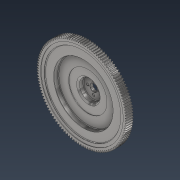
# Autodesk Inventor part: Koło zamachowe poprawione
Saved by Autodesk Inventor 2022 (Build 260153000, 153)
## iProperties
Created: 2023-05-24
Part Number: Koło zamachowe poprawione
Material: Generic
Document SubType Name: Modeling
Designer: wikto
Density: 1 g/cm^3
Appearance: Polished - Small Pyramid Knurl
Author: wikto
Autodesk Inventor part; units mm, degrees
ref_plane "YZ Plane" through (0, 0, 0) normal (1, 0, 0) x (0, 1, 0)
ref_plane "XZ Plane" through (0, 0, 0) normal (0, 1, 0) x (-1, 0, 0)
ref_plane "XY Plane" through (0, 0, 0) normal (0, 0, 1) x (1, 0, 0)
sketch "Sketch2" plane through (0, 0, 20) normal (0, 0, 1) x (0.9945, 0.1045, 0)
  arc A0 (6.9843, 152.34) -> (4.8056, 146.7964) centre (39.556, 136.339) ccw projected
  arc A1 (4.8056, 146.7964) -> (2.8837, 146.8467) centre (0, 0) ccw projected
  arc A2 (2.8837, 146.8467) -> (0.9981, 152.4967) centre (-32.3663, 138.2223) ccw projected
  arc A3 (0.9981, 152.4967) -> (-0.9981, 152.4967) centre (0, 0) ccw projected
  arc A4 (-0.9981, 152.4967) -> (-2.8837, 146.8467) centre (32.3663, 138.2223) ccw projected
  arc A5 (-2.8837, 146.8467) -> (-4.8056, 146.7964) centre (0, 0) ccw projected
  arc A6 (-4.8056, 146.7964) -> (-6.9843, 152.34) centre (-39.556, 136.339) ccw projected
  arc A7 (-6.9843, 152.34) -> (-8.9778, 152.2355) centre (0, 0) ccw projected
  arc A8 (-8.9778, 152.2355) -> (-10.5651, 146.4945) centre (25.088, 139.7268) ccw projected
  arc A9 (-10.5651, 146.4945) -> (-12.4818, 146.3437) centre (0, 0) ccw projected
  arc A10 (-12.4818, 146.3437) -> (-14.9476, 151.7657) centre (-46.6372, 134.0819) ccw projected
  arc A11 (-14.9476, 151.7657) -> (-16.9329, 151.557) centre (0, 0) ccw projected
  arc A12 (-16.9329, 151.557) -> (-18.2176, 145.7408) centre (17.7408, 140.8483) ccw projected
  arc A13 (-18.2176, 145.7408) -> (-20.1237, 145.4899) centre (0, 0) ccw projected
  arc A14 (-20.1237, 145.4899) -> (-22.8699, 150.7754) centre (-53.5906, 131.4574) ccw projected
  arc A15 (-22.8699, 150.7754) -> (-24.8416, 150.4631) centre (0, 0) ccw projected
  arc A16 (-24.8416, 150.4631) -> (-25.8201, 144.5877) centre (10.3451, 141.5838) ccw projected
  arc A17 (-25.8201, 144.5877) -> (-27.7105, 144.2373) centre (0, 0) ccw projected
  arc A18 (-27.7105, 144.2373) -> (-30.7296, 149.3718) centre (-60.3971, 128.4725) ccw projected
  arc A19 (-30.7296, 149.3718) -> (-32.6821, 148.9568) centre (0, 0) ccw projected
  arc A20 (-32.6821, 148.9568) -> (-33.3518, 143.0382) centre (2.921, 141.9312) ccw projected
  arc A21 (-33.3518, 143.0382) -> (-35.2213, 142.5894) centre (0, 0) ccw projected
  arc A22 (-35.2213, 142.5894) -> (-38.505, 147.5589) centre (-67.038, 125.1355) ccw projected
  arc A23 (-38.505, 147.5589) -> (-40.4332, 147.0422) centre (0, 0) ccw projected
  arc A24 (-40.4332, 147.0422) -> (-40.7922, 141.0967) centre (-4.5111, 141.8895) ccw projected
  arc A25 (-40.7922, 141.0967) -> (-42.6356, 140.5506) centre (0, 0) ccw projected
  arc A26 (-42.6356, 140.5506) -> (-46.1748, 145.3414) centre (-73.4952, 121.4555) ccw projected
  arc A27 (-46.1748, 145.3414) -> (-48.0733, 144.7246) centre (0, 0) ccw projected
  arc A28 (-48.0733, 144.7246) -> (-48.1207, 138.7684) centre (-11.9309, 141.459) ccw projected
  arc A29 (-48.1207, 138.7684) -> (-49.933, 138.1266) centre (0, 0) ccw projected
  arc A30 (-49.933, 138.1266) -> (-53.7181, 142.7257) centre (-79.751, 117.4426) ccw projected
  arc A31 (-53.7181, 142.7257) -> (-55.5818, 142.0103) centre (0, 0) ccw projected
  arc A32 (-55.5818, 142.0103) -> (-55.3173, 136.0598) centre (-19.3179, 140.6407) ccw projected
  arc A33 (-55.3173, 136.0598) -> (-57.0935, 135.324) centre (0, 0) ccw projected
  arc A34 (-57.0935, 135.324) -> (-61.1142, 139.7187) centre (-85.7882, 113.1078) ccw projected
  arc A35 (-61.1142, 139.7187) -> (-62.9378, 138.9067) centre (0, 0) ccw projected
  arc A36 (-62.9378, 138.9067) -> (-62.3623, 132.9782) centre (-26.652, 139.4369) ccw projected
  arc A37 (-62.3623, 132.9782) -> (-64.0976, 132.1505) centre (0, 0) ccw projected
  arc A38 (-64.0976, 132.1505) -> (-68.3428, 136.3287) centre (-91.5902, 108.463) ccw projected
  arc A39 (-68.3428, 136.3287) -> (-70.1214, 135.4225) centre (0, 0) ccw projected
  arc A40 (-70.1214, 135.4225) -> (-69.2364, 129.5322) centre (-33.913, 137.851) ccw projected
  arc A41 (-69.2364, 129.5322) -> (-70.926, 128.6148) centre (0, 0) ccw projected
  arc A42 (-70.926, 128.6148) -> (-75.384, 132.5651) centre (-97.1412, 103.5209) ccw projected
  arc A43 (-75.384, 132.5651) -> (-77.1127, 131.567) centre (0, 0) ccw projected
  arc A44 (-77.1127, 131.567) -> (-75.9207, 125.7311) centre (-41.0811, 135.8872) ccw projected
  arc A45 (-75.9207, 125.7311) -> (-77.56, 124.7266) centre (0, 0) ccw projected
  arc A46 (-77.56, 124.7266) -> (-82.2186, 128.4381) centre (-102.426, 98.295) ccw projected
  arc A47 (-82.2186, 128.4381) -> (-83.8928, 127.3509) centre (0, 0) ccw projected
  arc A48 (-83.8928, 127.3509) -> (-82.3969, 121.5854) centre (-48.1366, 133.551) ccw projected
  arc A49 (-82.3969, 121.5854) -> (-83.9814, 120.4965) centre (0, 0) ccw projected
  arc A50 (-83.9814, 120.4965) -> (-88.8278, 123.9591) centre (-107.4299, 92.7998) ccw projected
  arc A51 (-88.8278, 123.9591) -> (-90.4428, 122.7858) centre (0, 0) ccw projected
  arc A52 (-90.4428, 122.7858) -> (-88.6473, 117.1065) centre (-55.0601, 130.8487) ccw projected
  arc A53 (-88.6473, 117.1065) -> (-90.1726, 115.9361) centre (0, 0) ccw projected
  arc A54 (-90.1726, 115.9361) -> (-95.1936, 119.1403) centre (-112.1395, 87.0501) ccw projected
  arc A55 (-95.1936, 119.1403) -> (-96.745, 117.8841) centre (0, 0) ccw projected
  arc A56 (-96.745, 117.8841) -> (-94.6547, 112.3065) centre (-61.8328, 127.7877) ccw projected
  arc A57 (-94.6547, 112.3065) -> (-96.1166, 111.0579) centre (0, 0) ccw projected
  arc A58 (-96.1166, 111.0579) -> (-101.2985, 113.995) centre (-116.5417, 81.0619) ccw projected
  arc A59 (-101.2985, 113.995) -> (-102.782, 112.6593) centre (0, 0) ccw projected
  arc A60 (-102.782, 112.6593) -> (-100.4026, 107.1988) centre (-68.4359, 124.3765) ccw projected
  arc A61 (-100.4026, 107.1988) -> (-101.7972, 105.8754) centre (0, 0) ccw projected
  arc A62 (-101.7972, 105.8754) -> (-107.1257, 108.5372) centre (-120.6244, 74.8515) ccw projected
  arc A63 (-107.1257, 108.5372) -> (-108.5372, 107.1257) centre (0, 0) ccw projected
  arc A64 (-108.5372, 107.1257) -> (-105.8754, 101.7972) centre (-74.8515, 120.6244) ccw projected
  arc A65 (-105.8754, 101.7972) -> (-107.1988, 100.4026) centre (0, 0) ccw projected
  arc A66 (-107.1988, 100.4026) -> (-112.6593, 102.782) centre (-124.3765, 68.4359) ccw projected
  arc A67 (-112.6593, 102.782) -> (-113.995, 101.2985) centre (0, 0) ccw projected
  arc A68 (-113.995, 101.2985) -> (-111.0579, 96.1166) centre (-81.0619, 116.5417) ccw projected
  arc A69 (-111.0579, 96.1166) -> (-112.3065, 94.6547) centre (0, 0) ccw projected
  arc A70 (-112.3065, 94.6547) -> (-117.8841, 96.745) centre (-127.7877, 61.8328) ccw projected
  arc A71 (-117.8841, 96.745) -> (-119.1403, 95.1936) centre (0, 0) ccw projected
  arc A72 (-119.1403, 95.1936) -> (-115.9361, 90.1726) centre (-87.0501, 112.1395) ccw projected
  arc A73 (-115.9361, 90.1726) -> (-117.1065, 88.6473) centre (0, 0) ccw projected
  arc A74 (-117.1065, 88.6473) -> (-122.7858, 90.4428) centre (-130.8487, 55.0601) ccw projected
  arc A75 (-122.7858, 90.4428) -> (-123.9591, 88.8278) centre (0, 0) ccw projected
  arc A76 (-123.9591, 88.8278) -> (-120.4965, 83.9814) centre (-92.7998, 107.4299) ccw projected
  arc A77 (-120.4965, 83.9814) -> (-121.5854, 82.3969) centre (0, 0) ccw projected
  arc A78 (-121.5854, 82.3969) -> (-127.3509, 83.8928) centre (-133.551, 48.1366) ccw projected
  arc A79 (-127.3509, 83.8928) -> (-128.4381, 82.2186) centre (0, 0) ccw projected
  arc A80 (-128.4381, 82.2186) -> (-124.7266, 77.56) centre (-98.295, 102.426) ccw projected
  arc A81 (-124.7266, 77.56) -> (-125.7311, 75.9207) centre (0, 0) ccw projected
  arc A82 (-125.7311, 75.9207) -> (-131.567, 77.1127) centre (-135.8872, 41.0811) ccw projected
  arc A83 (-131.567, 77.1127) -> (-132.5651, 75.384) centre (0, 0) ccw projected
  arc A84 (-132.5651, 75.384) -> (-128.6148, 70.926) centre (-103.5209, 97.1412) ccw projected
  arc A85 (-128.6148, 70.926) -> (-129.5322, 69.2364) centre (0, 0) ccw projected
  arc A86 (-129.5322, 69.2364) -> (-135.4225, 70.1214) centre (-137.851, 33.913) ccw projected
  arc A87 (-135.4225, 70.1214) -> (-136.3287, 68.3428) centre (0, 0) ccw projected
  arc A88 (-136.3287, 68.3428) -> (-132.1505, 64.0976) centre (-108.463, 91.5902) ccw projected
  arc A89 (-132.1505, 64.0976) -> (-132.9782, 62.3623) centre (0, 0) ccw projected
  arc A90 (-132.9782, 62.3623) -> (-138.9067, 62.9378) centre (-139.4369, 26.652) ccw projected
  arc A91 (-138.9067, 62.9378) -> (-139.7187, 61.1142) centre (0, 0) ccw projected
  arc A92 (-139.7187, 61.1142) -> (-135.324, 57.0935) centre (-113.1078, 85.7882) ccw projected
  arc A93 (-135.324, 57.0935) -> (-136.0598, 55.3173) centre (0, 0) ccw projected
  arc A94 (-136.0598, 55.3173) -> (-142.0103, 55.5818) centre (-140.6407, 19.3179) ccw projected
  arc A95 (-142.0103, 55.5818) -> (-142.7257, 53.7181) centre (0, 0) ccw projected
  arc A96 (-142.7257, 53.7181) -> (-138.1266, 49.933) centre (-117.4426, 79.751) ccw projected
  arc A97 (-138.1266, 49.933) -> (-138.7684, 48.1207) centre (0, 0) ccw projected
  arc A98 (-138.7684, 48.1207) -> (-144.7246, 48.0733) centre (-141.459, 11.9309) ccw projected
  arc A99 (-144.7246, 48.0733) -> (-145.3414, 46.1748) centre (0, 0) ccw projected
  arc A100 (-145.3414, 46.1748) -> (-140.5506, 42.6356) centre (-121.4555, 73.4952) ccw projected
  arc A101 (-140.5506, 42.6356) -> (-141.0967, 40.7922) centre (0, 0) ccw projected
  arc A102 (-141.0967, 40.7922) -> (-147.0422, 40.4332) centre (-141.8895, 4.5111) ccw projected
  arc A103 (-147.0422, 40.4332) -> (-147.5589, 38.505) centre (0, 0) ccw projected
  arc A104 (-147.5589, 38.505) -> (-142.5894, 35.2213) centre (-125.1355, 67.038) ccw projected
  arc A105 (-142.5894, 35.2213) -> (-143.0382, 33.3518) centre (0, 0) ccw projected
  arc A106 (-143.0382, 33.3518) -> (-148.9568, 32.6821) centre (-141.9312, -2.921) ccw projected
  arc A107 (-148.9568, 32.6821) -> (-149.3718, 30.7296) centre (0, 0) ccw projected
  arc A108 (-149.3718, 30.7296) -> (-144.2373, 27.7105) centre (-128.4725, 60.3971) ccw projected
  arc A109 (-144.2373, 27.7105) -> (-144.5877, 25.8201) centre (0, 0) ccw projected
  arc A110 (-144.5877, 25.8201) -> (-150.4631, 24.8416) centre (-141.5838, -10.3451) ccw projected
  arc A111 (-150.4631, 24.8416) -> (-150.7754, 22.8699) centre (0, 0) ccw projected
  arc A112 (-150.7754, 22.8699) -> (-145.4899, 20.1237) centre (-131.4574, 53.5906) ccw projected
  arc A113 (-145.4899, 20.1237) -> (-145.7408, 18.2176) centre (0, 0) ccw projected
  arc A114 (-145.7408, 18.2176) -> (-151.557, 16.9329) centre (-140.8483, -17.7408) ccw projected
  arc A115 (-151.557, 16.9329) -> (-151.7657, 14.9476) centre (0, 0) ccw projected
  arc A116 (-151.7657, 14.9476) -> (-146.3437, 12.4818) centre (-134.0819, 46.6372) ccw projected
  arc A117 (-146.3437, 12.4818) -> (-146.4945, 10.5651) centre (0, 0) ccw projected
  arc A118 (-146.4945, 10.5651) -> (-152.2355, 8.9778) centre (-139.7268, -25.088) ccw projected
  arc A119 (-152.2355, 8.9778) -> (-152.34, 6.9843) centre (0, 0) ccw projected
  arc A120 (-152.34, 6.9843) -> (-146.7964, 4.8056) centre (-136.339, 39.556) ccw projected
  arc A121 (-146.7964, 4.8056) -> (-146.8467, 2.8837) centre (0, 0) ccw projected
  arc A122 (-146.8467, 2.8837) -> (-152.4967, 0.9981) centre (-138.2223, -32.3663) ccw projected
  arc A123 (-152.4967, 0.9981) -> (-152.4967, -0.9981) centre (0, 0) ccw projected
  arc A124 (-152.4967, -0.9981) -> (-146.8467, -2.8837) centre (-138.2223, 32.3663) ccw projected
  arc A125 (-146.8467, -2.8837) -> (-146.7964, -4.8056) centre (0, 0) ccw projected
  arc A126 (-146.7964, -4.8056) -> (-152.34, -6.9843) centre (-136.339, -39.556) ccw projected
  arc A127 (-152.34, -6.9843) -> (-152.2355, -8.9778) centre (0, 0) ccw projected
  arc A128 (-152.2355, -8.9778) -> (-146.4945, -10.5651) centre (-139.7268, 25.088) ccw projected
  arc A129 (-146.4945, -10.5651) -> (-146.3437, -12.4818) centre (0, 0) ccw projected
  arc A130 (-146.3437, -12.4818) -> (-151.7657, -14.9476) centre (-134.0819, -46.6372) ccw projected
  arc A131 (-151.7657, -14.9476) -> (-151.557, -16.9329) centre (0, 0) ccw projected
  arc A132 (-151.557, -16.9329) -> (-145.7408, -18.2176) centre (-140.8483, 17.7408) ccw projected
  arc A133 (-145.7408, -18.2176) -> (-145.4899, -20.1237) centre (0, 0) ccw projected
  arc A134 (-145.4899, -20.1237) -> (-150.7754, -22.8699) centre (-131.4574, -53.5906) ccw projected
  arc A135 (-150.7754, -22.8699) -> (-150.4631, -24.8416) centre (0, 0) ccw projected
  arc A136 (-150.4631, -24.8416) -> (-144.5877, -25.8201) centre (-141.5838, 10.3451) ccw projected
  arc A137 (-144.5877, -25.8201) -> (-144.2373, -27.7105) centre (0, 0) ccw projected
  arc A138 (-144.2373, -27.7105) -> (-149.3718, -30.7296) centre (-128.4725, -60.3971) ccw projected
  arc A139 (-149.3718, -30.7296) -> (-148.9568, -32.6821) centre (0, 0) ccw projected
  arc A140 (-148.9568, -32.6821) -> (-143.0382, -33.3518) centre (-141.9312, 2.921) ccw projected
  arc A141 (-143.0382, -33.3518) -> (-142.5894, -35.2213) centre (0, 0) ccw projected
  arc A142 (-142.5894, -35.2213) -> (-147.5589, -38.505) centre (-125.1355, -67.038) ccw projected
  arc A143 (-147.5589, -38.505) -> (-147.0422, -40.4332) centre (0, 0) ccw projected
  arc A144 (-147.0422, -40.4332) -> (-141.0967, -40.7922) centre (-141.8895, -4.5111) ccw projected
  arc A145 (-141.0967, -40.7922) -> (-140.5506, -42.6356) centre (0, 0) ccw projected
  arc A146 (-140.5506, -42.6356) -> (-145.3414, -46.1748) centre (-121.4555, -73.4952) ccw projected
  arc A147 (-145.3414, -46.1748) -> (-144.7246, -48.0733) centre (0, 0) ccw projected
  arc A148 (-144.7246, -48.0733) -> (-138.7684, -48.1207) centre (-141.459, -11.9309) ccw projected
  arc A149 (-138.7684, -48.1207) -> (-138.1266, -49.933) centre (0, 0) ccw projected
  arc A150 (-138.1266, -49.933) -> (-142.7257, -53.7181) centre (-117.4426, -79.751) ccw projected
  arc A151 (-142.7257, -53.7181) -> (-142.0103, -55.5818) centre (0, 0) ccw projected
  arc A152 (-142.0103, -55.5818) -> (-136.0598, -55.3173) centre (-140.6407, -19.3179) ccw projected
  arc A153 (-136.0598, -55.3173) -> (-135.324, -57.0935) centre (0, 0) ccw projected
  arc A154 (-135.324, -57.0935) -> (-139.7187, -61.1142) centre (-113.1078, -85.7882) ccw projected
  arc A155 (-139.7187, -61.1142) -> (-138.9067, -62.9378) centre (0, 0) ccw projected
  arc A156 (-138.9067, -62.9378) -> (-132.9782, -62.3623) centre (-139.4369, -26.652) ccw projected
  arc A157 (-132.9782, -62.3623) -> (-132.1505, -64.0976) centre (0, 0) ccw projected
  arc A158 (-132.1505, -64.0976) -> (-136.3287, -68.3428) centre (-108.463, -91.5902) ccw projected
  arc A159 (-136.3287, -68.3428) -> (-135.4225, -70.1214) centre (0, 0) ccw projected
  arc A160 (-135.4225, -70.1214) -> (-129.5322, -69.2364) centre (-137.851, -33.913) ccw projected
  arc A161 (-129.5322, -69.2364) -> (-128.6148, -70.926) centre (0, 0) ccw projected
  arc A162 (-128.6148, -70.926) -> (-132.5651, -75.384) centre (-103.5209, -97.1412) ccw projected
  arc A163 (-132.5651, -75.384) -> (-131.567, -77.1127) centre (0, 0) ccw projected
  arc A164 (-131.567, -77.1127) -> (-125.7311, -75.9207) centre (-135.8872, -41.0811) ccw projected
  arc A165 (-125.7311, -75.9207) -> (-124.7266, -77.56) centre (0, 0) ccw projected
  arc A166 (-124.7266, -77.56) -> (-128.4381, -82.2186) centre (-98.295, -102.426) ccw projected
  arc A167 (-128.4381, -82.2186) -> (-127.3509, -83.8928) centre (0, 0) ccw projected
  arc A168 (-127.3509, -83.8928) -> (-121.5854, -82.3969) centre (-133.551, -48.1366) ccw projected
  arc A169 (-121.5854, -82.3969) -> (-120.4965, -83.9814) centre (0, 0) ccw projected
  arc A170 (-120.4965, -83.9814) -> (-123.9591, -88.8278) centre (-92.7998, -107.4299) ccw projected
  arc A171 (-123.9591, -88.8278) -> (-122.7858, -90.4428) centre (0, 0) ccw projected
  arc A172 (-122.7858, -90.4428) -> (-117.1065, -88.6473) centre (-130.8487, -55.0601) ccw projected
  arc A173 (-117.1065, -88.6473) -> (-115.9361, -90.1726) centre (0, 0) ccw projected
  arc A174 (-115.9361, -90.1726) -> (-119.1403, -95.1936) centre (-87.0501, -112.1395) ccw projected
  arc A175 (-119.1403, -95.1936) -> (-117.8841, -96.745) centre (0, 0) ccw projected
  arc A176 (-117.8841, -96.745) -> (-112.3065, -94.6547) centre (-127.7877, -61.8328) ccw projected
  arc A177 (-112.3065, -94.6547) -> (-111.0579, -96.1166) centre (0, 0) ccw projected
  arc A178 (-111.0579, -96.1166) -> (-113.995, -101.2985) centre (-81.0619, -116.5417) ccw projected
  arc A179 (-113.995, -101.2985) -> (-112.6593, -102.782) centre (0, 0) ccw projected
  arc A180 (-112.6593, -102.782) -> (-107.1988, -100.4026) centre (-124.3765, -68.4359) ccw projected
  arc A181 (-107.1988, -100.4026) -> (-105.8754, -101.7972) centre (0, 0) ccw projected
  arc A182 (-105.8754, -101.7972) -> (-108.5372, -107.1257) centre (-74.8515, -120.6244) ccw projected
  arc A183 (-108.5372, -107.1257) -> (-107.1257, -108.5372) centre (0, 0) ccw projected
  arc A184 (-107.1257, -108.5372) -> (-101.7972, -105.8754) centre (-120.6244, -74.8515) ccw projected
  arc A185 (-101.7972, -105.8754) -> (-100.4026, -107.1988) centre (0, 0) ccw projected
  arc A186 (-100.4026, -107.1988) -> (-102.782, -112.6593) centre (-68.4359, -124.3765) ccw projected
  arc A187 (-102.782, -112.6593) -> (-101.2985, -113.995) centre (0, 0) ccw projected
  arc A188 (-101.2985, -113.995) -> (-96.1166, -111.0579) centre (-116.5417, -81.0619) ccw projected
  arc A189 (-96.1166, -111.0579) -> (-94.6547, -112.3065) centre (0, 0) ccw projected
  arc A190 (-94.6547, -112.3065) -> (-96.745, -117.8841) centre (-61.8328, -127.7877) ccw projected
  arc A191 (-96.745, -117.8841) -> (-95.1936, -119.1403) centre (0, 0) ccw projected
  arc A192 (-95.1936, -119.1403) -> (-90.1726, -115.9361) centre (-112.1395, -87.0501) ccw projected
  arc A193 (-90.1726, -115.9361) -> (-88.6473, -117.1065) centre (0, 0) ccw projected
  arc A194 (-88.6473, -117.1065) -> (-90.4428, -122.7858) centre (-55.0601, -130.8487) ccw projected
  arc A195 (-90.4428, -122.7858) -> (-88.8278, -123.9591) centre (0, 0) ccw projected
  arc A196 (-88.8278, -123.9591) -> (-83.9814, -120.4965) centre (-107.4299, -92.7998) ccw projected
  arc A197 (-83.9814, -120.4965) -> (-82.3969, -121.5854) centre (0, 0) ccw projected
  arc A198 (-82.3969, -121.5854) -> (-83.8928, -127.3509) centre (-48.1366, -133.551) ccw projected
  arc A199 (-83.8928, -127.3509) -> (-82.2186, -128.4381) centre (0, 0) ccw projected
  arc A200 (-82.2186, -128.4381) -> (-77.56, -124.7266) centre (-102.426, -98.295) ccw projected
  arc A201 (-77.56, -124.7266) -> (-75.9207, -125.7311) centre (0, 0) ccw projected
  arc A202 (-75.9207, -125.7311) -> (-77.1127, -131.567) centre (-41.0811, -135.8872) ccw projected
  arc A203 (-77.1127, -131.567) -> (-75.384, -132.5651) centre (0, 0) ccw projected
  arc A204 (-75.384, -132.5651) -> (-70.926, -128.6148) centre (-97.1412, -103.5209) ccw projected
  arc A205 (-70.926, -128.6148) -> (-69.2364, -129.5322) centre (0, 0) ccw projected
  arc A206 (-69.2364, -129.5322) -> (-70.1214, -135.4225) centre (-33.913, -137.851) ccw projected
  arc A207 (-70.1214, -135.4225) -> (-68.3428, -136.3287) centre (0, 0) ccw projected
  arc A208 (-68.3428, -136.3287) -> (-64.0976, -132.1505) centre (-91.5902, -108.463) ccw projected
  arc A209 (-64.0976, -132.1505) -> (-62.3623, -132.9782) centre (0, 0) ccw projected
  arc A210 (-62.3623, -132.9782) -> (-62.9378, -138.9067) centre (-26.652, -139.4369) ccw projected
  arc A211 (-62.9378, -138.9067) -> (-61.1142, -139.7187) centre (0, 0) ccw projected
  arc A212 (-61.1142, -139.7187) -> (-57.0935, -135.324) centre (-85.7882, -113.1078) ccw projected
  arc A213 (-57.0935, -135.324) -> (-55.3173, -136.0598) centre (0, 0) ccw projected
  arc A214 (-55.3173, -136.0598) -> (-55.5818, -142.0103) centre (-19.3179, -140.6407) ccw projected
  arc A215 (-55.5818, -142.0103) -> (-53.7181, -142.7257) centre (0, 0) ccw projected
  arc A216 (-53.7181, -142.7257) -> (-49.933, -138.1266) centre (-79.751, -117.4426) ccw projected
  arc A217 (-49.933, -138.1266) -> (-48.1207, -138.7684) centre (0, 0) ccw projected
  arc A218 (-48.1207, -138.7684) -> (-48.0733, -144.7246) centre (-11.9309, -141.459) ccw projected
  arc A219 (-48.0733, -144.7246) -> (-46.1748, -145.3414) centre (0, 0) ccw projected
  arc A220 (-46.1748, -145.3414) -> (-42.6356, -140.5506) centre (-73.4952, -121.4555) ccw projected
  arc A221 (-42.6356, -140.5506) -> (-40.7922, -141.0967) centre (0, 0) ccw projected
  arc A222 (-40.7922, -141.0967) -> (-40.4332, -147.0422) centre (-4.5111, -141.8895) ccw projected
  arc A223 (-40.4332, -147.0422) -> (-38.505, -147.5589) centre (0, 0) ccw projected
  arc A224 (-38.505, -147.5589) -> (-35.2213, -142.5894) centre (-67.038, -125.1355) ccw projected
  arc A225 (-35.2213, -142.5894) -> (-33.3518, -143.0382) centre (0, 0) ccw projected
  arc A226 (-33.3518, -143.0382) -> (-32.6821, -148.9568) centre (2.921, -141.9312) ccw projected
  arc A227 (-32.6821, -148.9568) -> (-30.7296, -149.3718) centre (0, 0) ccw projected
  arc A228 (-30.7296, -149.3718) -> (-27.7105, -144.2373) centre (-60.3971, -128.4725) ccw projected
  arc A229 (-27.7105, -144.2373) -> (-25.8201, -144.5877) centre (0, 0) ccw projected
  arc A230 (-25.8201, -144.5877) -> (-24.8416, -150.4631) centre (10.3451, -141.5838) ccw projected
  arc A231 (-24.8416, -150.4631) -> (-22.8699, -150.7754) centre (0, 0) ccw projected
  arc A232 (-22.8699, -150.7754) -> (-20.1237, -145.4899) centre (-53.5906, -131.4574) ccw projected
  arc A233 (-20.1237, -145.4899) -> (-18.2176, -145.7408) centre (0, 0) ccw projected
  arc A234 (-18.2176, -145.7408) -> (-16.9329, -151.557) centre (17.7408, -140.8483) ccw projected
  arc A235 (-16.9329, -151.557) -> (-14.9476, -151.7657) centre (0, 0) ccw projected
  arc A236 (-14.9476, -151.7657) -> (-12.4818, -146.3437) centre (-46.6372, -134.0819) ccw projected
  arc A237 (-12.4818, -146.3437) -> (-10.5651, -146.4945) centre (0, 0) ccw projected
  arc A238 (-10.5651, -146.4945) -> (-8.9778, -152.2355) centre (25.088, -139.7268) ccw projected
  arc A239 (-8.9778, -152.2355) -> (-6.9843, -152.34) centre (0, 0) ccw projected
  arc A240 (-6.9843, -152.34) -> (-4.8056, -146.7964) centre (-39.556, -136.339) ccw projected
  arc A241 (-4.8056, -146.7964) -> (-2.8837, -146.8467) centre (0, 0) ccw projected
  arc A242 (-2.8837, -146.8467) -> (-0.9981, -152.4967) centre (32.3663, -138.2223) ccw projected
  arc A243 (-0.9981, -152.4967) -> (0.9981, -152.4967) centre (0, 0) ccw projected
  arc A244 (0.9981, -152.4967) -> (2.8837, -146.8467) centre (-32.3663, -138.2223) ccw projected
  arc A245 (2.8837, -146.8467) -> (4.8056, -146.7964) centre (0, 0) ccw projected
  arc A246 (4.8056, -146.7964) -> (6.9843, -152.34) centre (39.556, -136.339) ccw projected
  arc A247 (6.9843, -152.34) -> (8.9778, -152.2355) centre (0, 0) ccw projected
  arc A248 (8.9778, -152.2355) -> (10.5651, -146.4945) centre (-25.088, -139.7268) ccw projected
  arc A249 (10.5651, -146.4945) -> (12.4818, -146.3437) centre (0, 0) ccw projected
  arc A250 (12.4818, -146.3437) -> (14.9476, -151.7657) centre (46.6372, -134.0819) ccw projected
  arc A251 (14.9476, -151.7657) -> (16.9329, -151.557) centre (0, 0) ccw projected
  arc A252 (16.9329, -151.557) -> (18.2176, -145.7408) centre (-17.7408, -140.8483) ccw projected
  arc A253 (18.2176, -145.7408) -> (20.1237, -145.4899) centre (0, 0) ccw projected
  arc A254 (20.1237, -145.4899) -> (22.8699, -150.7754) centre (53.5906, -131.4574) ccw projected
  arc A255 (22.8699, -150.7754) -> (24.8416, -150.4631) centre (0, 0) ccw projected
  arc A256 (24.8416, -150.4631) -> (25.8201, -144.5877) centre (-10.3451, -141.5838) ccw projected
  arc A257 (25.8201, -144.5877) -> (27.7105, -144.2373) centre (0, 0) ccw projected
  arc A258 (27.7105, -144.2373) -> (30.7296, -149.3718) centre (60.3971, -128.4725) ccw projected
  arc A259 (30.7296, -149.3718) -> (32.6821, -148.9568) centre (0, 0) ccw projected
  arc A260 (32.6821, -148.9568) -> (33.3518, -143.0382) centre (-2.921, -141.9312) ccw projected
  arc A261 (33.3518, -143.0382) -> (35.2213, -142.5894) centre (0, 0) ccw projected
  arc A262 (35.2213, -142.5894) -> (38.505, -147.5589) centre (67.038, -125.1355) ccw projected
  arc A263 (38.505, -147.5589) -> (40.4332, -147.0422) centre (0, 0) ccw projected
  arc A264 (40.4332, -147.0422) -> (40.7922, -141.0967) centre (4.5111, -141.8895) ccw projected
  arc A265 (40.7922, -141.0967) -> (42.6356, -140.5506) centre (0, 0) ccw projected
  arc A266 (42.6356, -140.5506) -> (46.1748, -145.3414) centre (73.4952, -121.4555) ccw projected
  arc A267 (46.1748, -145.3414) -> (48.0733, -144.7246) centre (0, 0) ccw projected
  arc A268 (48.0733, -144.7246) -> (48.1207, -138.7684) centre (11.9309, -141.459) ccw projected
  arc A269 (48.1207, -138.7684) -> (49.933, -138.1266) centre (0, 0) ccw projected
  arc A270 (49.933, -138.1266) -> (53.7181, -142.7257) centre (79.751, -117.4426) ccw projected
  arc A271 (53.7181, -142.7257) -> (55.5818, -142.0103) centre (0, 0) ccw projected
  arc A272 (55.5818, -142.0103) -> (55.3173, -136.0598) centre (19.3179, -140.6407) ccw projected
  arc A273 (55.3173, -136.0598) -> (57.0935, -135.324) centre (0, 0) ccw projected
  arc A274 (57.0935, -135.324) -> (61.1142, -139.7187) centre (85.7882, -113.1078) ccw projected
  arc A275 (61.1142, -139.7187) -> (62.9378, -138.9067) centre (0, 0) ccw projected
  arc A276 (62.9378, -138.9067) -> (62.3623, -132.9782) centre (26.652, -139.4369) ccw projected
  arc A277 (62.3623, -132.9782) -> (64.0976, -132.1505) centre (0, 0) ccw projected
  arc A278 (64.0976, -132.1505) -> (68.3428, -136.3287) centre (91.5902, -108.463) ccw projected
  arc A279 (68.3428, -136.3287) -> (70.1214, -135.4225) centre (0, 0) ccw projected
  arc A280 (70.1214, -135.4225) -> (69.2364, -129.5322) centre (33.913, -137.851) ccw projected
  arc A281 (69.2364, -129.5322) -> (70.926, -128.6148) centre (0, 0) ccw projected
  arc A282 (70.926, -128.6148) -> (75.384, -132.5651) centre (97.1412, -103.5209) ccw projected
  arc A283 (75.384, -132.5651) -> (77.1127, -131.567) centre (0, 0) ccw projected
  arc A284 (77.1127, -131.567) -> (75.9207, -125.7311) centre (41.0811, -135.8872) ccw projected
  arc A285 (75.9207, -125.7311) -> (77.56, -124.7266) centre (0, 0) ccw projected
  arc A286 (77.56, -124.7266) -> (82.2186, -128.4381) centre (102.426, -98.295) ccw projected
  arc A287 (82.2186, -128.4381) -> (83.8928, -127.3509) centre (0, 0) ccw projected
  arc A288 (83.8928, -127.3509) -> (82.3969, -121.5854) centre (48.1366, -133.551) ccw projected
  arc A289 (82.3969, -121.5854) -> (83.9814, -120.4965) centre (0, 0) ccw projected
  arc A290 (83.9814, -120.4965) -> (88.8278, -123.9591) centre (107.4299, -92.7998) ccw projected
  arc A291 (88.8278, -123.9591) -> (90.4428, -122.7858) centre (0, 0) ccw projected
  arc A292 (90.4428, -122.7858) -> (88.6473, -117.1065) centre (55.0601, -130.8487) ccw projected
  arc A293 (88.6473, -117.1065) -> (90.1726, -115.9361) centre (0, 0) ccw projected
  arc A294 (90.1726, -115.9361) -> (95.1936, -119.1403) centre (112.1395, -87.0501) ccw projected
  arc A295 (95.1936, -119.1403) -> (96.745, -117.8841) centre (0, 0) ccw projected
  arc A296 (96.745, -117.8841) -> (94.6547, -112.3065) centre (61.8328, -127.7877) ccw projected
  arc A297 (94.6547, -112.3065) -> (96.1166, -111.0579) centre (0, 0) ccw projected
  arc A298 (96.1166, -111.0579) -> (101.2985, -113.995) centre (116.5417, -81.0619) ccw projected
  arc A299 (101.2985, -113.995) -> (102.782, -112.6593) centre (0, 0) ccw projected
  arc A300 (102.782, -112.6593) -> (100.4026, -107.1988) centre (68.4359, -124.3765) ccw projected
  arc A301 (100.4026, -107.1988) -> (101.7972, -105.8754) centre (0, 0) ccw projected
  arc A302 (101.7972, -105.8754) -> (107.1257, -108.5372) centre (120.6244, -74.8515) ccw projected
  arc A303 (107.1257, -108.5372) -> (108.5372, -107.1257) centre (0, 0) ccw projected
  arc A304 (108.5372, -107.1257) -> (105.8754, -101.7972) centre (74.8515, -120.6244) ccw projected
  arc A305 (105.8754, -101.7972) -> (107.1988, -100.4026) centre (0, 0) ccw projected
  arc A306 (107.1988, -100.4026) -> (112.6593, -102.782) centre (124.3765, -68.4359) ccw projected
  arc A307 (112.6593, -102.782) -> (113.995, -101.2985) centre (0, 0) ccw projected
  arc A308 (113.995, -101.2985) -> (111.0579, -96.1166) centre (81.0619, -116.5417) ccw projected
  arc A309 (111.0579, -96.1166) -> (112.3065, -94.6547) centre (0, 0) ccw projected
  arc A310 (112.3065, -94.6547) -> (117.8841, -96.745) centre (127.7877, -61.8328) ccw projected
  arc A311 (117.8841, -96.745) -> (119.1403, -95.1936) centre (0, 0) ccw projected
  arc A312 (119.1403, -95.1936) -> (115.9361, -90.1726) centre (87.0501, -112.1395) ccw projected
  arc A313 (115.9361, -90.1726) -> (117.1065, -88.6473) centre (0, 0) ccw projected
  arc A314 (117.1065, -88.6473) -> (122.7858, -90.4428) centre (130.8487, -55.0601) ccw projected
  arc A315 (122.7858, -90.4428) -> (123.9591, -88.8278) centre (0, 0) ccw projected
  arc A316 (123.9591, -88.8278) -> (120.4965, -83.9814) centre (92.7998, -107.4299) ccw projected
  arc A317 (120.4965, -83.9814) -> (121.5854, -82.3969) centre (0, 0) ccw projected
  arc A318 (121.5854, -82.3969) -> (127.3509, -83.8928) centre (133.551, -48.1366) ccw projected
  arc A319 (127.3509, -83.8928) -> (128.4381, -82.2186) centre (0, 0) ccw projected
  arc A320 (128.4381, -82.2186) -> (124.7266, -77.56) centre (98.295, -102.426) ccw projected
  arc A321 (124.7266, -77.56) -> (125.7311, -75.9207) centre (0, 0) ccw projected
  arc A322 (125.7311, -75.9207) -> (131.567, -77.1127) centre (135.8872, -41.0811) ccw projected
  arc A323 (131.567, -77.1127) -> (132.5651, -75.384) centre (0, 0) ccw projected
  arc A324 (132.5651, -75.384) -> (128.6148, -70.926) centre (103.5209, -97.1412) ccw projected
  arc A325 (128.6148, -70.926) -> (129.5322, -69.2364) centre (0, 0) ccw projected
  arc A326 (129.5322, -69.2364) -> (135.4225, -70.1214) centre (137.851, -33.913) ccw projected
  arc A327 (135.4225, -70.1214) -> (136.3287, -68.3428) centre (0, 0) ccw projected
  arc A328 (136.3287, -68.3428) -> (132.1505, -64.0976) centre (108.463, -91.5902) ccw projected
  arc A329 (132.1505, -64.0976) -> (132.9782, -62.3623) centre (0, 0) ccw projected
  arc A330 (132.9782, -62.3623) -> (138.9067, -62.9378) centre (139.4369, -26.652) ccw projected
  arc A331 (138.9067, -62.9378) -> (139.7187, -61.1142) centre (0, 0) ccw projected
  arc A332 (139.7187, -61.1142) -> (135.324, -57.0935) centre (113.1078, -85.7882) ccw projected
  arc A333 (135.324, -57.0935) -> (136.0598, -55.3173) centre (0, 0) ccw projected
  arc A334 (136.0598, -55.3173) -> (142.0103, -55.5818) centre (140.6407, -19.3179) ccw projected
  arc A335 (142.0103, -55.5818) -> (142.7257, -53.7181) centre (0, 0) ccw projected
  arc A336 (142.7257, -53.7181) -> (138.1266, -49.933) centre (117.4426, -79.751) ccw projected
  arc A337 (138.1266, -49.933) -> (138.7684, -48.1207) centre (0, 0) ccw projected
  arc A338 (138.7684, -48.1207) -> (144.7246, -48.0733) centre (141.459, -11.9309) ccw projected
  arc A339 (144.7246, -48.0733) -> (145.3414, -46.1748) centre (0, 0) ccw projected
  arc A340 (145.3414, -46.1748) -> (140.5506, -42.6356) centre (121.4555, -73.4952) ccw projected
  arc A341 (140.5506, -42.6356) -> (141.0967, -40.7922) centre (0, 0) ccw projected
  arc A342 (141.0967, -40.7922) -> (147.0422, -40.4332) centre (141.8895, -4.5111) ccw projected
  arc A343 (147.0422, -40.4332) -> (147.5589, -38.505) centre (0, 0) ccw projected
  arc A344 (147.5589, -38.505) -> (142.5894, -35.2213) centre (125.1355, -67.038) ccw projected
  arc A345 (142.5894, -35.2213) -> (143.0382, -33.3518) centre (0, 0) ccw projected
  arc A346 (143.0382, -33.3518) -> (148.9568, -32.6821) centre (141.9312, 2.921) ccw projected
  arc A347 (148.9568, -32.6821) -> (149.3718, -30.7296) centre (0, 0) ccw projected
  arc A348 (149.3718, -30.7296) -> (144.2373, -27.7105) centre (128.4725, -60.3971) ccw projected
  arc A349 (144.2373, -27.7105) -> (144.5877, -25.8201) centre (0, 0) ccw projected
  arc A350 (144.5877, -25.8201) -> (150.4631, -24.8416) centre (141.5838, 10.3451) ccw projected
  arc A351 (150.4631, -24.8416) -> (150.7754, -22.8699) centre (0, 0) ccw projected
  arc A352 (150.7754, -22.8699) -> (145.4899, -20.1237) centre (131.4574, -53.5906) ccw projected
  arc A353 (145.4899, -20.1237) -> (145.7408, -18.2176) centre (0, 0) ccw projected
  arc A354 (145.7408, -18.2176) -> (151.557, -16.9329) centre (140.8483, 17.7408) ccw projected
  arc A355 (151.557, -16.9329) -> (151.7657, -14.9476) centre (0, 0) ccw projected
  arc A356 (151.7657, -14.9476) -> (146.3437, -12.4818) centre (134.0819, -46.6372) ccw projected
  arc A357 (146.3437, -12.4818) -> (146.4945, -10.5651) centre (0, 0) ccw projected
  arc A358 (146.4945, -10.5651) -> (152.2355, -8.9778) centre (139.7268, 25.088) ccw projected
  arc A359 (152.2355, -8.9778) -> (152.34, -6.9843) centre (0, 0) ccw projected
  arc A360 (152.34, -6.9843) -> (146.7964, -4.8056) centre (136.339, -39.556) ccw projected
  arc A361 (146.7964, -4.8056) -> (146.8467, -2.8837) centre (0, 0) ccw projected
  arc A362 (146.8467, -2.8837) -> (152.4967, -0.9981) centre (138.2223, 32.3663) ccw projected
  arc A363 (152.4967, -0.9981) -> (152.4967, 0.9981) centre (0, 0) ccw projected
  arc A364 (152.4967, 0.9981) -> (146.8467, 2.8837) centre (138.2223, -32.3663) ccw projected
  arc A365 (146.8467, 2.8837) -> (146.7964, 4.8056) centre (0, 0) ccw projected
  arc A366 (146.7964, 4.8056) -> (152.34, 6.9843) centre (136.339, 39.556) ccw projected
  arc A367 (152.34, 6.9843) -> (152.2355, 8.9778) centre (0, 0) ccw projected
  arc A368 (152.2355, 8.9778) -> (146.4945, 10.5651) centre (139.7268, -25.088) ccw projected
  arc A369 (146.4945, 10.5651) -> (146.3437, 12.4818) centre (0, 0) ccw projected
  arc A370 (146.3437, 12.4818) -> (151.7657, 14.9476) centre (134.0819, 46.6372) ccw projected
  arc A371 (151.7657, 14.9476) -> (151.557, 16.9329) centre (0, 0) ccw projected
  arc A372 (151.557, 16.9329) -> (145.7408, 18.2176) centre (140.8483, -17.7408) ccw projected
  arc A373 (145.7408, 18.2176) -> (145.4899, 20.1237) centre (0, 0) ccw projected
  arc A374 (145.4899, 20.1237) -> (150.7754, 22.8699) centre (131.4574, 53.5906) ccw projected
  arc A375 (150.7754, 22.8699) -> (150.4631, 24.8416) centre (0, 0) ccw projected
  arc A376 (150.4631, 24.8416) -> (144.5877, 25.8201) centre (141.5838, -10.3451) ccw projected
  arc A377 (144.5877, 25.8201) -> (144.2373, 27.7105) centre (0, 0) ccw projected
  arc A378 (144.2373, 27.7105) -> (149.3718, 30.7296) centre (128.4725, 60.3971) ccw projected
  arc A379 (149.3718, 30.7296) -> (148.9568, 32.6821) centre (0, 0) ccw projected
  arc A380 (148.9568, 32.6821) -> (143.0382, 33.3518) centre (141.9312, -2.921) ccw projected
  arc A381 (143.0382, 33.3518) -> (142.5894, 35.2213) centre (0, 0) ccw projected
  arc A382 (142.5894, 35.2213) -> (147.5589, 38.505) centre (125.1355, 67.038) ccw projected
  arc A383 (147.5589, 38.505) -> (147.0422, 40.4332) centre (0, 0) ccw projected
  arc A384 (147.0422, 40.4332) -> (141.0967, 40.7922) centre (141.8895, 4.5111) ccw projected
  arc A385 (141.0967, 40.7922) -> (140.5506, 42.6356) centre (0, 0) ccw projected
  arc A386 (140.5506, 42.6356) -> (145.3414, 46.1748) centre (121.4555, 73.4952) ccw projected
  arc A387 (145.3414, 46.1748) -> (144.7246, 48.0733) centre (0, 0) ccw projected
  arc A388 (144.7246, 48.0733) -> (138.7684, 48.1207) centre (141.459, 11.9309) ccw projected
  arc A389 (138.7684, 48.1207) -> (138.1266, 49.933) centre (0, 0) ccw projected
  arc A390 (138.1266, 49.933) -> (142.7257, 53.7181) centre (117.4426, 79.751) ccw projected
  arc A391 (142.7257, 53.7181) -> (142.0103, 55.5818) centre (0, 0) ccw projected
  arc A392 (142.0103, 55.5818) -> (136.0598, 55.3173) centre (140.6407, 19.3179) ccw projected
  arc A393 (136.0598, 55.3173) -> (135.324, 57.0935) centre (0, 0) ccw projected
  arc A394 (135.324, 57.0935) -> (139.7187, 61.1142) centre (113.1078, 85.7882) ccw projected
  arc A395 (139.7187, 61.1142) -> (138.9067, 62.9378) centre (0, 0) ccw projected
  arc A396 (138.9067, 62.9378) -> (132.9782, 62.3623) centre (139.4369, 26.652) ccw projected
  arc A397 (132.9782, 62.3623) -> (132.1505, 64.0976) centre (0, 0) ccw projected
  arc A398 (132.1505, 64.0976) -> (136.3287, 68.3428) centre (108.463, 91.5902) ccw projected
  arc A399 (136.3287, 68.3428) -> (135.4225, 70.1214) centre (0, 0) ccw projected
  arc A400 (135.4225, 70.1214) -> (129.5322, 69.2364) centre (137.851, 33.913) ccw projected
  arc A401 (129.5322, 69.2364) -> (128.6148, 70.926) centre (0, 0) ccw projected
  arc A402 (128.6148, 70.926) -> (132.5651, 75.384) centre (103.5209, 97.1412) ccw projected
  arc A403 (132.5651, 75.384) -> (131.567, 77.1127) centre (0, 0) ccw projected
  arc A404 (131.567, 77.1127) -> (125.7311, 75.9207) centre (135.8872, 41.0811) ccw projected
  arc A405 (125.7311, 75.9207) -> (124.7266, 77.56) centre (0, 0) ccw projected
  arc A406 (124.7266, 77.56) -> (128.4381, 82.2186) centre (98.295, 102.426) ccw projected
  arc A407 (128.4381, 82.2186) -> (127.3509, 83.8928) centre (0, 0) ccw projected
  arc A408 (127.3509, 83.8928) -> (121.5854, 82.3969) centre (133.551, 48.1366) ccw projected
  arc A409 (121.5854, 82.3969) -> (120.4965, 83.9814) centre (0, 0) ccw projected
  arc A410 (120.4965, 83.9814) -> (123.9591, 88.8278) centre (92.7998, 107.4299) ccw projected
  arc A411 (123.9591, 88.8278) -> (122.7858, 90.4428) centre (0, 0) ccw projected
  arc A412 (122.7858, 90.4428) -> (117.1065, 88.6473) centre (130.8487, 55.0601) ccw projected
  arc A413 (117.1065, 88.6473) -> (115.9361, 90.1726) centre (0, 0) ccw projected
  arc A414 (115.9361, 90.1726) -> (119.1403, 95.1936) centre (87.0501, 112.1395) ccw projected
  arc A415 (119.1403, 95.1936) -> (117.8841, 96.745) centre (0, 0) ccw projected
  arc A416 (117.8841, 96.745) -> (112.3065, 94.6547) centre (127.7877, 61.8328) ccw projected
  arc A417 (112.3065, 94.6547) -> (111.0579, 96.1166) centre (0, 0) ccw projected
  arc A418 (111.0579, 96.1166) -> (113.995, 101.2985) centre (81.0619, 116.5417) ccw projected
  arc A419 (113.995, 101.2985) -> (112.6593, 102.782) centre (0, 0) ccw projected
  arc A420 (112.6593, 102.782) -> (107.1988, 100.4026) centre (124.3765, 68.4359) ccw projected
  arc A421 (107.1988, 100.4026) -> (105.8754, 101.7972) centre (0, 0) ccw projected
  arc A422 (105.8754, 101.7972) -> (108.5372, 107.1257) centre (74.8515, 120.6244) ccw projected
  arc A423 (108.5372, 107.1257) -> (107.1257, 108.5372) centre (0, 0) ccw projected
  arc A424 (107.1257, 108.5372) -> (101.7972, 105.8754) centre (120.6244, 74.8515) ccw projected
  arc A425 (101.7972, 105.8754) -> (100.4026, 107.1988) centre (0, 0) ccw projected
  arc A426 (100.4026, 107.1988) -> (102.782, 112.6593) centre (68.4359, 124.3765) ccw projected
  arc A427 (102.782, 112.6593) -> (101.2985, 113.995) centre (0, 0) ccw projected
  arc A428 (101.2985, 113.995) -> (96.1166, 111.0579) centre (116.5417, 81.0619) ccw projected
  arc A429 (96.1166, 111.0579) -> (94.6547, 112.3065) centre (0, 0) ccw projected
  arc A430 (94.6547, 112.3065) -> (96.745, 117.8841) centre (61.8328, 127.7877) ccw projected
  arc A431 (96.745, 117.8841) -> (95.1936, 119.1403) centre (0, 0) ccw projected
  arc A432 (95.1936, 119.1403) -> (90.1726, 115.9361) centre (112.1395, 87.0501) ccw projected
  arc A433 (90.1726, 115.9361) -> (88.6473, 117.1065) centre (0, 0) ccw projected
  arc A434 (88.6473, 117.1065) -> (90.4428, 122.7858) centre (55.0601, 130.8487) ccw projected
  arc A435 (90.4428, 122.7858) -> (88.8278, 123.9591) centre (0, 0) ccw projected
  arc A436 (88.8278, 123.9591) -> (83.9814, 120.4965) centre (107.4299, 92.7998) ccw projected
  arc A437 (83.9814, 120.4965) -> (82.3969, 121.5854) centre (0, 0) ccw projected
  arc A438 (82.3969, 121.5854) -> (83.8928, 127.3509) centre (48.1366, 133.551) ccw projected
  arc A439 (83.8928, 127.3509) -> (82.2186, 128.4381) centre (0, 0) ccw projected
  arc A440 (82.2186, 128.4381) -> (77.56, 124.7266) centre (102.426, 98.295) ccw projected
  arc A441 (77.56, 124.7266) -> (75.9207, 125.7311) centre (0, 0) ccw projected
  arc A442 (75.9207, 125.7311) -> (77.1127, 131.567) centre (41.0811, 135.8872) ccw projected
  arc A443 (77.1127, 131.567) -> (75.384, 132.5651) centre (0, 0) ccw projected
  arc A444 (75.384, 132.5651) -> (70.926, 128.6148) centre (97.1412, 103.5209) ccw projected
  arc A445 (70.926, 128.6148) -> (69.2364, 129.5322) centre (0, 0) ccw projected
  arc A446 (69.2364, 129.5322) -> (70.1214, 135.4225) centre (33.913, 137.851) ccw projected
  arc A447 (70.1214, 135.4225) -> (68.3428, 136.3287) centre (0, 0) ccw projected
  arc A448 (68.3428, 136.3287) -> (64.0976, 132.1505) centre (91.5902, 108.463) ccw projected
  arc A449 (64.0976, 132.1505) -> (62.3623, 132.9782) centre (0, 0) ccw projected
  arc A450 (62.3623, 132.9782) -> (62.9378, 138.9067) centre (26.652, 139.4369) ccw projected
  arc A451 (62.9378, 138.9067) -> (61.1142, 139.7187) centre (0, 0) ccw projected
  arc A452 (61.1142, 139.7187) -> (57.0935, 135.324) centre (85.7882, 113.1078) ccw projected
  arc A453 (57.0935, 135.324) -> (55.3173, 136.0598) centre (0, 0) ccw projected
  arc A454 (55.3173, 136.0598) -> (55.5818, 142.0103) centre (19.3179, 140.6407) ccw projected
  arc A455 (55.5818, 142.0103) -> (53.7181, 142.7257) centre (0, 0) ccw projected
  arc A456 (53.7181, 142.7257) -> (49.933, 138.1266) centre (79.751, 117.4426) ccw projected
  arc A457 (49.933, 138.1266) -> (48.1207, 138.7684) centre (0, 0) ccw projected
  arc A458 (48.1207, 138.7684) -> (48.0733, 144.7246) centre (11.9309, 141.459) ccw projected
  arc A459 (48.0733, 144.7246) -> (46.1748, 145.3414) centre (0, 0) ccw projected
  arc A460 (46.1748, 145.3414) -> (42.6356, 140.5506) centre (73.4952, 121.4555) ccw projected
  arc A461 (42.6356, 140.5506) -> (40.7922, 141.0967) centre (0, 0) ccw projected
  arc A462 (40.7922, 141.0967) -> (40.4332, 147.0422) centre (4.5111, 141.8895) ccw projected
  arc A463 (40.4332, 147.0422) -> (38.505, 147.5589) centre (0, 0) ccw projected
  arc A464 (38.505, 147.5589) -> (35.2213, 142.5894) centre (67.038, 125.1355) ccw projected
  arc A465 (35.2213, 142.5894) -> (33.3518, 143.0382) centre (0, 0) ccw projected
  arc A466 (33.3518, 143.0382) -> (32.6821, 148.9568) centre (-2.921, 141.9312) ccw projected
  arc A467 (32.6821, 148.9568) -> (30.7296, 149.3718) centre (0, 0) ccw projected
  arc A468 (30.7296, 149.3718) -> (27.7105, 144.2373) centre (60.3971, 128.4725) ccw projected
  arc A469 (27.7105, 144.2373) -> (25.8201, 144.5877) centre (0, 0) ccw projected
  arc A470 (25.8201, 144.5877) -> (24.8416, 150.4631) centre (-10.3451, 141.5838) ccw projected
  arc A471 (24.8416, 150.4631) -> (22.8699, 150.7754) centre (0, 0) ccw projected
  arc A472 (22.8699, 150.7754) -> (20.1237, 145.4899) centre (53.5906, 131.4574) ccw projected
  arc A473 (20.1237, 145.4899) -> (18.2176, 145.7408) centre (0, 0) ccw projected
  arc A474 (18.2176, 145.7408) -> (16.9329, 151.557) centre (-17.7408, 140.8483) ccw projected
  arc A475 (16.9329, 151.557) -> (14.9476, 151.7657) centre (0, 0) ccw projected
  arc A476 (14.9476, 151.7657) -> (12.4818, 146.3437) centre (46.6372, 134.0819) ccw projected
  arc A477 (12.4818, 146.3437) -> (10.5651, 146.4945) centre (0, 0) ccw projected
  arc A478 (10.5651, 146.4945) -> (8.9778, 152.2355) centre (-25.088, 139.7268) ccw projected
  arc A479 (8.9778, 152.2355) -> (6.9843, 152.34) centre (0, 0) ccw projected
extrude "Extrusion1" add sketch "Sketch2" against normal blind 50
sketch "Sketch1" plane through (0, 0, 20) normal (0, 0, 1) x (0.9945, 0.1045, 0)
  circle A0 centre (0, 0) radius 140
  circle A1 centre (0, 0) radius 130
  circle A2 centre (0, 0) radius 100
  circle A3 centre (0, 0) radius 65
  circle A4 centre (0, 0) radius 35
  circle A5 centre (0, 0) radius 14.15
  dimension "d1" = 280
  dimension "d2" = 260
  dimension "d3" = 200
  dimension "d4" = 28.3
  dimension "d5" = 70
  dimension "d6" = 130
  constraints: 6 centre point, 6 coincident
  measures "d1" diameter of A0
  measures "d2" diameter of A1
  measures "d3" diameter of A2
  measures "d4" diameter of A5
  measures "d5" diameter of A4
  measures "d6" diameter of A3
extrude "Extrusion2" cut sketch "Sketch1" against normal blind 2 contours A0 | A1 | A2 | A3 | A4 | A5
extrude "Extrusion3" cut sketch "Sketch1" against normal blind 5 contours A1 | A2 | A3 | A4 | A5
extrude "Extrusion4" cut sketch "Sketch1" against normal blind 20 contours A2 | A3 | A4 | A5
extrude "Extrusion5" cut sketch "Sketch1" against normal blind 22 contours A3 | A4 | A5
extrude "Extrusion6" cut sketch "Sketch1" against normal through all contours A5
extrude "Extrusion7" cut sketch "Sketch1" against normal blind 40 contours A4 | A5
sketch "Sketch3" plane through (0, 0, -20) normal (0, 0, 1) x (1, 0, 0)
  circle A0 centre (0, 0) radius 20.5
  point P0 (0, 20.5)
  point P1 (-20.5, 0)
  point P2 (0, -20.5)
  point P3 (20.5, 0)
  dimension "d21" = 41
  dimension "d24" = 360
  constraints: 2 vertical alignment, 1 coincident, 7 other
hole "Hole1" at (0, 20.5, -20) at (-20.5, 0, -20) at (0, -20.5, -20) at (20.5, 0, -20) direction (0, 0, -1) diameter 8 end through all
chamfer "Chamfer1" distance 5 angle 45 1 edges at (-34.8083, -3.6585, -2)
fillet "Fillet1" radius 2 3 edges at (-34.8083, -3.6585, -20) (-99.4522, -10.4528, 0) (-129.2878, -13.5887, 15)
chamfer "Chamfer2" distance 1 angle 45 1 edges at (-99.4522, -10.4528, 15)
sketch "Sketch4" plane through (0, 0, -30) normal (0, 0, -1) x (-0.9945, -0.1045, 0)
  circle A0 centre (0, 0) radius 27.5
  circle A1 centre (0, 0) radius 35
  dimension "d40" = 55
  dimension "d41" = 70
  constraints: 2 centre point, 2 coincident
  measures "d40" diameter of A0
  measures "d41" diameter of A1
extrude "Extrusion8" add sketch "Sketch4" along normal blind 5
sketch "Sketch5" plane through (0, 0, -30) normal (0, 0, -1) x (-0.9945, -0.1045, 0)
  circle A0 centre (0, 0) radius 35 projected
  circle A1 centre (0, 0) radius 140 projected
  circle A2 centre (0, 0) radius 14.15 projected
  circle A3 centre (0, 0) radius 155
  circle A4 centre (0, 0) radius 127.5
  circle A5 centre (0, 0) radius 75
  circle A6 centre (0, 0) radius 12.5
  dimension "d44" = 310
  dimension "d45" = 255
  dimension "d46" = 150
  dimension "d61" = 25
  constraints: 4 centre point, 4 coincident
  measures "d44" diameter of A3
  measures "d45" diameter of A4
  measures "d46" diameter of A5
  measures "d61" diameter of A6
extrude "Extrusion9" cut sketch "Sketch5" against normal blind 11 contours A5
extrude "Extrusion10" cut sketch "Sketch5" against normal blind 14 contours A4
extrude "Extrusion11" cut sketch "Sketch5" against normal blind 30 contours A1
extrude "Extrusion12" cut sketch "Sketch5" against normal blind 28 contours A3
fillet "Fillet2" radius 7 1 edges at (126.8015, 13.3274, -16)
fillet "Fillet3" radius 1 5 edges at (74.5891, 7.8396, -16) (74.5891, 7.8396, -19) (34.8083, 3.6585, -35) (27.3494, 2.8745, -35) (27.3494, 2.8745, -30)
fillet "Fillet4" radius 4 1 edges at (34.8083, 3.6585, -19)
extrude "Extrusion13" add sketch "Sketch5" against normal up to surface (10 mm away) contours A2
chamfer "Chamfer3" distance 0.5 angle 45 10 edges at (0, -16.5, -30) (20.5, 4, -30) (-20.5, 4, -30) (0, 24.5, -30) (0, -16.5, -20) (20.5, 4, -20) (-20.5, 4, -20) (0, 24.5, -20) (12.4315, 1.3066, -20) (12.4315, 1.3066, -30)
body "Solid1"
